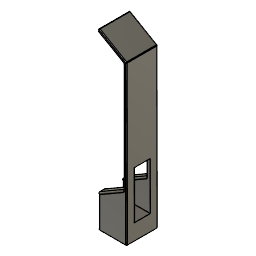
cable-slot (Autodesk Fusion 360 design; units mm, degrees)
part number: 2026-07-22-15-00-25-850
Autodesk Fusion 360 part; units mm, degrees
sketch "Sketch1" plane through (0, 0, 0) normal (0, 1, 0) x (1, 0, 0)
  line L0 (0, 0) -> (18, 0)
  line L1 (0, -110) -> (17.8218, -99.7106)
  line L2 (0, -110) -> (20.5788, -110) construction
  line L3 (0, -20) -> (20.0578, -20) construction
  line L4 (16, -98.453) -> (16, -29.2376)
  line L5 (0, -107.6906) -> (16, -98.453)
  line L6 (17.8218, -99.7106) -> (18, 0)
  line L7 (0, -20) -> (16, -29.2376)
  line L8 (0, -20) -> (0, 0)
  line L9 (0, -107.6906) -> (0, -110)
  dimension "d1" = 18
  dimension "d2" = 110
  dimension "d3" = 30
  dimension "d4" = 2
  dimension "d7" = 20
  dimension "d9" = 20.5788
  dimension "d10" = 9.2376
  dimension "d11" = 20.0578
  constraint horizontal L0
  constraint coincident L0.start L8.end
  constraint horizontal L2
  constraint horizontal L3
  constraint equal L1 L2
  constraint perpendicular L0 L8
  constraint perpendicular L2 L9
  constraint parallel L1 L5
  constraint parallel L4 L9
  constraint collinear L8 L9
  constraint equal L5 L7
  measures "d1" distance of L0.start L0.end
  measures "d2" distance of L0.start L1.start
  measures "d3" angle of L1 L2
  measures "d4" distance of L1 L5.start
  measures "d7" distance of L0 L3
  measures "d9" distance of L1.start L1.end
  measures "d10" distance of L3 L4.end
  measures "d11" distance of L3.end L8
extrude "Extrude1" add sketch "Sketch1" along normal blind 19.85
sketch "Sketch2" plane through (17.9999, 0, 0.0322) normal (0.999998, 0, 0.001788) x (0, 1, 0)
  line L0 (0, 99.6786) -> (0, -0.0322)
  line L1 (0, -0.0322) -> (19.85, -0.0322)
  line L2 (19.85, -0.0322) -> (19.85, 99.6786)
  line L3 (19.85, 99.6786) -> (0, 99.6786)
  line L4 (15, 40) -> (5, 40)
  line L5 (5, 40) -> (5, 10)
  line L6 (5, 10) -> (15, 10)
  line L7 (15, 10) -> (15, 40)
  line L8 (15, 40) -> (5, 10) construction
  line L9 (5, 40) -> (15, 10) construction
  point P0 (10, 25)
  dimension "d14" = 15
  dimension "d15" = 5
  dimension "d16" = 5
  dimension "d17" = 10.0322
  constraint horizontal L4
  constraint perpendicular L4 L5
  constraint parallel L4 L6
  constraint parallel L5 L7
  constraint coincident L8 P0
  constraint coincident L9 P0
  measures "d14" distance of L6 P0
  measures "d15" distance of L5 P0
  measures "d16" distance of L0 L5
  measures "d17" distance of L1 L6
extrude "Extrude2" cut sketch "Sketch2" against normal blind 50 contours L4 L5 L6 L7
fillet "Fillet1" radius 0.5 14 edges at (8.9109, 0, 104.8553) (8, 0, 103.0718) (0, 9.925, 110) (8.9109, 19.85, 104.8553) (17.8218, 9.925, 99.7106) (17.9109, 0, 49.8553) (16, 0, 63.8453) (0, 9.925, 107.6906) (8, 19.85, 103.0718) (16, 9.925, 98.453) (17.9109, 19.85, 49.8553) (16, 19.85, 63.8453) (0, 19.85, 108.8453) (0, 0, 108.8453)
fillet "Fillet2" radius 1 9 edges at (8.25, 19.85, 24.7631) (8, 15, 24.6188) (8, 5, 24.6188) (8.25, 0, 24.7631) (0, 15, 15) (0, 5, 15) (0, 19.85, 10) (0, 0, 10) (0, 10, 10)
